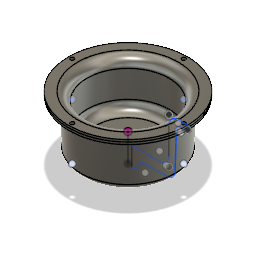
3dprintsensorholder (v1~recovered) (Autodesk Fusion 360 design; units mm, degrees)
Autodesk Fusion 360 part; units mm, degrees
sketch "Sketch2" plane through (0, 0, 0) normal (0, 0, 1) x (1, 0, 0)
  line L0 (0, 0) -> (0, -30)
  line L1 (4, -31.1432) -> (4, -11.1432)
  line L2 (4, -11.1432) -> (34, -11.1432)
  line L3 (44, -1.1432) -> (44, 27.8196)
  line L4 (54, 37.8196) -> (64, 37.8196)
  arc A0 (34, -11.1432) -> (44, -1.1432) centre (34, -1.1432) ccw
  arc A1 (54, 37.8196) -> (44, 27.8196) centre (54, 27.8196) ccw
  line L5 (64, 37.8196) -> (64, 35.5267)
  arc A2 (43.4913, -20.6081) -> (50.659, -13.6222) centre (41.0324, -10.9151) ccw
  arc A3 (63.6266, 32.8196) -> (64, 35.5267) centre (54, 35.5267) ccw
  line L6 (4, -31.1432) -> (9.934, -31.1432)
  line L7 (9.934, -31.1432) -> (9.934, -29.1081)
  line L8 (18.434, -20.6081) -> (43.4913, -20.6081)
  arc A4 (18.434, -20.6081) -> (9.934, -29.1081) centre (18.434, -29.1081) ccw
  line L9 (63.6266, 32.8196) -> (56.881, 32.8196)
  line L10 (51.8832, 27.9668) -> (50.659, -13.6222)
  arc A5 (56.881, 32.8196) -> (51.8832, 27.9668) centre (56.881, 27.8196) ccw
  point P0 (44, -11.1432)
  point P1 (44, 37.8196)
  point P2 (64, 33.8196)
  dimension "d1" = 30
  dimension "d2" = 4
  dimension "d3" = 20
  dimension "d4" = 40
  dimension "d5" = 20
  dimension "d6" = 10
  dimension "d7" = 4
  dimension "d8" = 10
  dimension "d9" = 8.5
  dimension "d10" = 5
  dimension "d18" = 5
  dimension "d19" = 50.659
  dimension "d20" = 20
  measures "d1" distance of L0.start L0.end
  measures "d2" distance of L0 L1
  measures "d3" distance of L1.start L1.end
  measures "d4" distance of L1.end P0
  measures "d5" distance of P1 L4.end
  measures "d6" radius of A0
  measures "d7" distance of L4.end P2
  measures "d8" radius of A2
  measures "d9" radius of A4
  measures "d10" radius of A5
  measures "d18" distance of L4 L9
  measures "d19" distance of L0 A2.end
  measures "d20" distance of L1.start L1.end
revolve "Revolve1" add sketch "Sketch2" angle 360 about axis through (0, 0, 0) along (0, -1, 0)
sketch "Sketch3" plane through (0, 0, 0) normal (0, 1, 0) x (1, 0, 0)
  circle A0 centre (60, 0) radius 2
  circle A1 centre (0, 60) radius 2
  circle A2 centre (-60, 0) radius 2
  circle A3 centre (0, -60) radius 2
  dimension "d12" = 4
  dimension "d13" = 60
  dimension "d15" = 360
  measures "d12" diameter of A0
  measures "d13" distance of origin A0.centre
extrude "Extrude1" cut sketch "Sketch3" along normal blind 100
